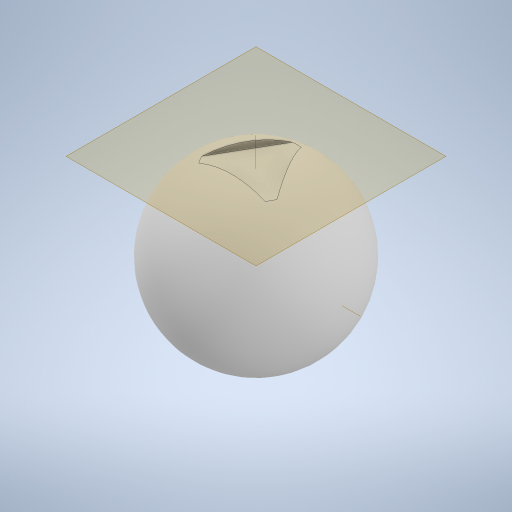
# Autodesk Inventor part: D20
Saved by Autodesk Inventor 2023 (Build 270158030, 158C)
## iProperties
Created: 2024-01-29
Part Number: D20
Material: Generic
Document SubType Name: Modeling
Designer: Imogen Heard
Density: 1 g/cm^3
Appearance: Default
Author: Imogen Heard
Autodesk Inventor part; units mm, degrees
sketch "Sketch1" plane through (0, 0, 0) normal (0, 0, 1) x (1, 0, 0)
  circle A0 centre (0, 0) radius 25
  line L0 (0, 29.9302) -> (0, -28.7192)
  point P0 (0, 25)
  point P1 (0, -25)
  dimension "d0" = 50
  constraints: 2 end point, 2 vertical alignment, 1 centre point, 1 coincident
  measures "d0" diameter of A0
revolve "Revolution1" add sketch "Sketch1" angle 360 about axis through (0, 29.9302, 0) along (0, -1, 0) picked at (6.5153, 5.1957) contours A0 L0
ref_plane "Work Plane16" through (0, 25, 0) normal (0, 1, 0) x (-1, 0, 0)
sketch "Sketch3" plane through (0, 25, 0) normal (0, 1, 0) x (-1, 0, 0)
  line L0 (12.1244, 7) -> (0, -14)
  line L1 (0, -14) -> (-12.1244, 7)
  line L2 (-12.1244, 7) -> (12.1244, 7)
  line L3 (35, 0) -> (-35, 0) projected
  point P0 (0, 0)
  point P1 (0, 0)
  dimension "d16" = 7
  constraints: 6 end point, 1 coincident, 1 parallel, 7 other
  measures "d16" distance from line of L2 point (0, 0)
extrude "Extrusion2" cut sketch "Sketch3" against normal blind 3
sketch "Sketch2" plane through (0, 0, 0) normal (1, 0, 0) x (0, 1, 0)
  line L0 (46.5152, 12.5741) -> (33.9411, 0)
  line L1 (33.9411, 0) -> (0, 33.9411)
  line L2 (0, 33.9411) -> (12.5741, 46.5152)
  line L3 (12.5741, 46.5152) -> (46.5152, 12.5741)
  circle A0 centre (0, 0) radius 25 projected
  line L4 (0, -36.1422) -> (0, 41.8532) projected
  point P0 (12.0208, 21.9203)
  point P1 (21.9203, 12.0208)
  dimension "d2" = 24
  dimension "d3" = 45
  dimension "d4" = 0
  constraints: 8 end point, 2 parallel, 1 perpendicular, 1 vertical alignment
  measures "d2" distance from line of L1 A0.centre
  measures "d3" angle of L4 L1
  measures "d4" vertical distance of point (0, 0) L0.end
body "Solid1"
